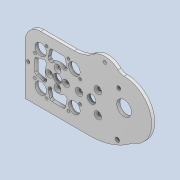
# Autodesk Inventor part: アームモータマウント
Saved by Autodesk Inventor 2020.4 (Build 244396000, 396)
## iProperties
Created: 2021-04-23
Part Number: アームモータマウント
Material: アルミニウム 2014-T4
Document SubType Name: Modeling
Designer: happy
Density: 2.8 g/cm^3
Appearance: サテン
Mass: 49.3876 g
Surface Area: 145.773 cm^2
Volume: 17.6384 cm^3
Author: happy
Autodesk Inventor part; units mm, degrees
ref_plane "YZ Plane" through (0, 0, 0) normal (1, 0, 0) x (0, 1, 0)
ref_plane "XZ Plane" through (0, 0, 0) normal (0, 1, 0) x (-1, 0, 0)
ref_plane "XY Plane" through (0, 0, 0) normal (0, 0, 1) x (1, 0, 0)
sketch "スケッチ1" plane through (0, 0, 0) normal (0, 0, 1) x (1, 0, 0)
  circle A0 centre (80.0196, 33.6804) radius 15
  circle A1 centre (112.2, 33.6804) radius 15
  circle A2 centre (112.2, 1.5) radius 15 construction
  circle A3 centre (80.0196, 1.5) radius 15 construction
  circle A4 centre (96.1098, 17.5902) radius 3.5 construction
  circle A5 centre (80.0196, 33.6804) radius 5.5
  circle A6 centre (112.2, 33.6804) radius 5.5
  circle A7 centre (80.0196, 1.5) radius 5.5
  circle A8 centre (112.2, 1.5) radius 5.5
  circle A9 centre (96.1098, 17.5902) radius 4.025
  circle A10 centre (74.3628, 28.0235) radius 1.3
  circle A11 centre (85.6765, 39.3372) radius 1.3
  circle A12 centre (106.5431, 39.3372) radius 1.3
  circle A13 centre (117.8569, 28.0235) radius 1.3
  circle A14 centre (117.8569, 7.1569) radius 1.3
  circle A15 centre (106.5431, -4.1569) radius 1.3
  circle A16 centre (85.6765, -4.1569) radius 1.3
  circle A17 centre (74.3628, 7.1569) radius 1.3
  line L0 (85.6765, 39.3372) -> (74.3628, 28.0235) construction
  line L1 (74.3628, 7.1569) -> (85.6765, -4.1569) construction
  line L2 (106.5431, -4.1569) -> (117.8569, 7.1569) construction
  line L3 (117.8569, 28.0235) -> (106.5431, 39.3372) construction
  line L4 (80.0196, 33.6804) -> (96.1098, 17.5902) construction
  line L5 (96.1098, 17.5902) -> (112.2, 33.6804) construction
  line L6 (112.2, 1.5) -> (96.1098, 17.5902) construction
  line L7 (80.0196, 1.5) -> (96.1098, 17.5902) construction
  circle A18 centre (74.3628, 28.0235) radius 3.3
  circle A19 centre (80.0196, 33.6804) radius 7.5
  circle A20 centre (85.6765, 39.3372) radius 3.3
  circle A21 centre (106.5431, 39.3372) radius 3.3
  circle A22 centre (112.2, 33.6804) radius 7.5
  circle A23 centre (117.8569, 28.0235) radius 3.3
  circle A24 centre (117.8569, 7.1569) radius 3.3
  circle A25 centre (112.2, 1.5) radius 7.5
  circle A26 centre (106.5431, -4.1569) radius 3.3
  circle A27 centre (85.6765, -4.1569) radius 3.3
  circle A28 centre (80.0196, 1.5) radius 7.5
  circle A29 centre (74.3628, 7.1569) radius 3.3
  line L8 (72.7217, 35.4098) -> (71.1517, 28.7845)
  line L9 (75.1237, 24.8125) -> (81.749, 26.3825)
  line L10 (87.3175, 31.951) -> (88.8875, 38.5763)
  line L11 (84.9155, 42.5483) -> (78.2902, 40.9783)
  line L12 (107.3041, 42.5483) -> (113.9294, 40.9783)
  line L13 (119.4979, 35.4098) -> (121.0679, 28.7845)
  line L14 (117.0959, 24.8125) -> (110.4706, 26.3825)
  line L15 (104.9021, 31.951) -> (103.3321, 38.5763)
  line L16 (121.0679, 6.3959) -> (119.4979, -0.2294)
  line L17 (110.4706, 8.7979) -> (117.0959, 10.3679)
  line L18 (104.9021, 3.2294) -> (103.3321, -3.3959)
  line L19 (113.9294, -5.7979) -> (107.3041, -7.3679)
  line L20 (71.1517, 6.3959) -> (72.7217, -0.2294)
  line L21 (78.2902, -5.7979) -> (84.9155, -7.3679)
  line L22 (88.8875, -3.3959) -> (87.3175, 3.2294)
  line L23 (81.749, 8.7979) -> (75.1237, 10.3679)
  circle A30 centre (96.1098, 25.6116) radius 3 construction
  circle A31 centre (104.1312, 17.5902) radius 3 construction
  circle A32 centre (96.1098, 9.5688) radius 3 construction
  circle A33 centre (88.0884, 17.5902) radius 3 construction
  circle A34 centre (96.1098, 25.6116) radius 1.25
  circle A35 centre (88.0884, 17.5902) radius 1.25
  circle A36 centre (96.1098, 9.5688) radius 1.25
  circle A37 centre (104.1312, 17.5902) radius 1.25
  circle A38 centre (96.1098, 17.5902) radius 12.0214
  circle A39 centre (96.1098, 25.6116) radius 4 construction
  line L24 (80.0196, 33.6804) -> (112.2, 33.6804) construction
  line L25 (112.2, 1.5) -> (112.2, 33.6804) construction
  line L26 (80.0196, 33.6804) -> (80.0196, 1.5) construction
  line L27 (80.0196, 1.5) -> (112.2, 1.5) construction
  line L28 (80.0196, 48.6804) -> (112.2, 48.6804)
  line L29 (127.2, 33.6804) -> (127.2, -14.5)
  line L30 (127.2, -14.5) -> (65.0196, -14.5)
  line L31 (65.0196, -14.5) -> (65.0196, 33.6804)
  line L32 (83, -14.5) -> (133, -14.5) construction
  line L33 (117.8569, 39.3372) -> (74.3628, 39.3372)
  line L34 (74.3628, 39.3372) -> (74.3628, -4.1569)
  line L35 (74.3628, -4.1569) -> (117.8569, -4.1569)
  line L36 (117.8569, -4.1569) -> (117.8569, 39.3372)
  line L37 (83.7167, 27.1549) -> (86.3137, 24.5579)
  line L38 (89.1421, 27.3863) -> (86.5451, 29.9833)
  line L39 (105.6745, 29.9833) -> (103.0775, 27.3863)
  line L40 (108.503, 27.1549) -> (105.9059, 24.5579)
  line L41 (108.503, 8.0255) -> (105.9059, 10.6225)
  line L42 (105.6745, 5.197) -> (103.0775, 7.7941)
  line L43 (83.7167, 8.0255) -> (86.3137, 10.6225)
  line L44 (86.5451, 5.197) -> (89.1421, 7.7941)
  circle A40 centre (96.1098, 45.6804) radius 3 construction
  circle A41 centre (68.0196, 17.5902) radius 3 construction
  circle A42 centre (68.0196, 17.5902) radius 1.5
  circle A43 centre (96.1098, 45.6804) radius 1.5
  line L45 (127.2, 33.6804) -> (127.2, -14.5) construction
  line L46 (83, -14.5) -> (133, -14.5) construction
  circle A44 centre (128.7687, 16.8502) radius 6.025 construction
  circle A45 centre (160, 25) radius 2
  circle A46 centre (154.8697, 39.0954) radius 1.75
  circle A47 centre (128.7687, 16.8502) radius 4.025
  arc A48 (112.2, 48.6804) -> (130.0806, 54.5913) centre (112.2, 78.6804) ccw
  arc A49 (153.3164, 53.0826) -> (130.0806, 54.5913) centre (140.809, 40.1379) ccw
  arc A50 (153.3164, 53.0826) -> (160, 50.3812) centre (160, 60) ccw
  arc A51 (168.6809, 1.1495) -> (160, 50.3812) centre (160, 25) ccw
  arc A52 (168.6809, 1.1495) -> (165.807, -0.5048) centre (171.9707, -7.8892) ccw
  arc A53 (127.2, -14.5) -> (165.807, -0.5048) centre (127.2, 45.748) ccw
  circle A54 centre (134.7937, 27.2858) radius 1.5
  circle A55 centre (116.7187, 16.8502) radius 1.5
  circle A56 centre (134.7937, 6.4146) radius 1.5
  circle A57 centre (160, 25) radius 7.025
  line L47 (65.0196, -14.5) -> (65.0196, 33.6804)
  circle A58 centre (80.0196, 33.6804) radius 15 construction
  line L48 (80.0196, 48.6804) -> (112.2, 48.6804)
  circle A59 centre (112.2, 33.6804) radius 15 construction
  line L49 (127.2, -14.5) -> (65.0196, -14.5)
  circle A60 centre (80.0196, 33.6804) radius 3.05 construction
  circle A61 centre (112.2, 33.6804) radius 3.05 construction
  circle A62 centre (112.2, 1.5) radius 3.05 construction
  circle A63 centre (80.0196, 1.5) radius 3.05 construction
  circle A64 centre (96.1098, 17.5902) radius 2.85 construction
  circle A65 centre (128.7687, 16.8502) radius 5.7 construction
  circle A66 centre (160, 25) radius 21.5 construction
  circle A67 centre (128.7687, 16.8502) radius 28.5 construction
  circle A68 centre (128.7687, 16.8502) radius 29.4672 construction
  circle A69 centre (160, 25) radius 25.8772 construction
  circle A70 centre (80.0196, 33.6804) radius 6
  circle A71 centre (112.2, 33.6804) radius 6
  circle A72 centre (80.0196, 1.5) radius 6
  circle A73 centre (112.2, 1.5) radius 6
  arc A74 (112.2, 48.6804) -> (130.3338, 54.7813) centre (112.2, 78.6804) ccw
  arc A75 (153.6832, 53.4235) -> (160, 50.8812) centre (160, 60) ccw
  arc A76 (153.6832, 53.4235) -> (130.3338, 54.7813) centre (141.2141, 40.4419) ccw
  circle A77 centre (96.1098, 17.5902) radius 9.025
  circle A78 centre (128.7687, 16.8502) radius 6.025
  circle A79 centre (160, 25) radius 2
  arc A80 (168.8519, 0.6796) -> (160, 50.8812) centre (160, 25) ccw
  arc A81 (168.8519, 0.6796) -> (166.2672, -0.7743) centre (171.9707, -7.8892) ccw
  circle A82 centre (171.9707, -7.8892) radius 8.6188 construction
  arc A83 (127.2, -14.5) -> (166.2672, -0.7743) centre (127.2, 47.9609) ccw
  circle A84 centre (160, 60) radius 8.6188 construction
  circle A85 centre (154.8697, 39.0954) radius 3 construction
  circle A86 centre (154.8697, 39.0954) radius 1.75
  arc A87 (158.348, 26.1273) -> (99.1742, 26.079) centre (128.7687, 16.8502) ccw construction
  arc A88 (98.7866, 8.9713) -> (159.1095, 23.2092) centre (128.7687, 16.8502) ccw construction
  arc A89 (80.0196, 48.6804) -> (65.0196, 33.6804) centre (80.0196, 33.6804) ccw
  line L50 (65.0196, -14.5) -> (65.0196, 33.6804)
  circle A90 centre (80.0196, 33.6804) radius 15 construction
  line L51 (80.0196, 48.6804) -> (112.2, 48.6804)
  circle A91 centre (112.2, 33.6804) radius 15 construction
  line L52 (127.2, -14.5) -> (65.0196, -14.5)
  circle A92 centre (80.0196, 33.6804) radius 3.05 construction
  circle A93 centre (112.2, 33.6804) radius 3.05 construction
  circle A94 centre (112.2, 1.5) radius 3.05 construction
  circle A95 centre (80.0196, 1.5) radius 3.05 construction
  circle A96 centre (96.1098, 17.5902) radius 2.85 construction
  circle A97 centre (128.7687, 16.8502) radius 5.7 construction
  circle A98 centre (160, 25) radius 21.5 construction
  circle A99 centre (128.7687, 16.8502) radius 28.5 construction
  circle A100 centre (128.7687, 16.8502) radius 29.4672 construction
  circle A101 centre (160, 25) radius 25.8772 construction
  circle A102 centre (80.0196, 33.6804) radius 6
  circle A103 centre (112.2, 33.6804) radius 6
  circle A104 centre (80.0196, 1.5) radius 6
  circle A105 centre (112.2, 1.5) radius 6
  arc A106 (112.2, 48.6804) -> (130.5847, 54.9738) centre (112.2, 78.6804) ccw
  arc A107 (154.0473, 53.767) -> (160, 51.3812) centre (160, 60) ccw
  arc A108 (154.0473, 53.767) -> (130.5847, 54.9738) centre (141.6155, 40.7498) ccw
  circle A109 centre (96.1098, 17.5902) radius 9.025
  circle A110 centre (128.7687, 16.8502) radius 6.025
  circle A111 centre (160, 25) radius 2
  arc A112 (169.0229, 0.2098) -> (160, 51.3812) centre (160, 25) ccw
  arc A113 (169.0229, 0.2098) -> (166.7152, -1.0582) centre (171.9707, -7.8892) ccw
  circle A114 centre (171.9707, -7.8892) radius 8.6188 construction
  arc A115 (127.2, -14.5) -> (166.7152, -1.0582) centre (127.2, 50.3027) ccw
  circle A116 centre (160, 60) radius 8.6188 construction
  circle A117 centre (154.8697, 39.0954) radius 3 construction
  circle A118 centre (154.8697, 39.0954) radius 1.75
  arc A119 (158.348, 26.1273) -> (99.1742, 26.079) centre (128.7687, 16.8502) ccw construction
  arc A120 (98.7866, 8.9713) -> (159.1094, 23.2092) centre (128.7687, 16.8502) ccw construction
  arc A121 (80.0196, 48.6804) -> (65.0196, 33.6804) centre (80.0196, 33.6804) ccw
  circle A122 centre (141.6155, 53.7498) radius 5 construction
  circle A123 centre (141.6155, 53.7498) radius 3.2
  circle A124 centre (141.6155, 53.7498) radius 1.5
  circle A125 centre (153.5524, -4.4926) radius 2
  circle A126 centre (153.5524, -4.4926) radius 4 construction
  point P0 (0, 0)
  point P1 (0, 0)
  point P2 (117.8569, 24.7235)
  point P3 (117.8569, 10.4569)
  point P4 (103.2431, -4.1569)
  point P5 (88.9765, -4.1569)
  point P6 (88.9765, 39.3372)
  point P7 (103.2431, 39.3372)
  point P8 (74.3628, 10.4569)
  point P9 (74.3628, 24.7235)
  point P10 (167.1721, 0.4471)
  point P11 (0, 0)
  point P12 (96.1924, 17.5902)
  point P13 (80.1022, 1.5)
  point P14 (112.2826, 1.5)
  point P15 (112.2826, 33.6804)
  point P16 (80.1022, 33.6804)
  point P17 (160, 60)
  point P18 (147.9041, -10.9688)
  point P19 (0, 0)
  point P20 (96.1924, 17.5902)
  point P21 (80.1022, 1.5)
  point P22 (112.2826, 1.5)
  point P23 (112.2826, 33.6804)
  point P24 (80.1022, 33.6804)
  point P25 (160, 60)
  point P26 (148.0694, -11.0476)
  point P27 (130.3338, 54.7813)
  dimension "d0" = 11
  dimension "d1" = 2.6
  dimension "d2" = 16
  dimension "d3" = 2
  dimension "d4" = 2
  dimension "d5" = 2
  dimension "d6" = 8.05
  dimension "d7" = 6
  dimension "d8" = 2.5
  dimension "d9" = 8
  dimension "d10" = 4
  dimension "d11" = 4
  dimension "d12" = 4
  dimension "d13" = 4
  dimension "d14" = 6
  dimension "d15" = 6
  dimension "d16" = 3
  dimension "d17" = 3
  dimension "d21" = 8.05
  dimension "d22" = 3
  dimension "d36" = 14.05
  dimension "d38" = 12
  dimension "d39" = 30
  dimension "d40" = 18.05
  dimension "d41" = 12.05
  dimension "d42" = 4
  dimension "d43" = 0.5
  dimension "d44" = 18
  dimension "d45" = 3.5
  dimension "d46" = 31
  dimension "d47" = 62.4609
  dimension "d48" = 12
  dimension "d49" = 30
  dimension "d50" = 18.05
  dimension "d51" = 12.05
  dimension "d52" = 4
  dimension "d53" = 0
  dimension "d54" = 18
  dimension "d55" = 3.5
  dimension "d56" = 31
  dimension "d57" = 64.8027
  dimension "d58" = 10
  dimension "d59" = 6.4
  dimension "d60" = 3
  dimension "d68" = 4
  dimension "d69" = 8
  constraints: 122 centre point, 106 end point, 103 point on circle, 64 tangent, 40 coincident, 36 equal radius, 9 parallel, 6 concentric, 5 perpendicular, 5 vertical alignment, 4 horizontal, 4 midpoint, 3 equal length, 2 point on line, 2 vertical, 1 horizontal alignment, 50 other
  measures "d0" diameter of A5
  measures "d1" diameter of A10
  measures "d2" distance of L0.start L0.end
  measures "d3" radial gap between concentric circles of A10 A18
  measures "d4" radial gap between concentric circles of A5 A19
  measures "d5" radial gap between concentric circles of A11 A20
  measures "d6" diameter of A9
  measures "d7" diameter of A30
  measures "d8" diameter of A34
  measures "d9" diameter of A39
  measures "d10" distance between parallel lines of L37 L38
  measures "d11" distance between parallel lines of L40 L39
  measures "d12" distance between parallel lines of L42 L41
  measures "d13" distance between parallel lines of L44 L43
  measures "d14" diameter of A40
  measures "d15" diameter of A41
  measures "d16" diameter of A42
  measures "d17" diameter of A43
  measures "d21" diameter of A47
  measures "d22" diameter of A54
  measures "d36" diameter of A57
  measures "d38" diameter of A71
  measures "d39" radius of A74
  measures "d40" diameter of A77
  measures "d41" diameter of A78
  measures "d42" diameter of A79
  measures "d43" radial gap between concentric circles of A82 A81
  measures "d44" radius of A76
  measures "d45" diameter of A86
  measures "d46" radius of A87
  measures "d47" radius of A83
  measures "d48" diameter of A103
  measures "d49" radius of A106
  measures "d50" diameter of A109
  measures "d51" diameter of A110
  measures "d52" diameter of A111
  measures "d53" radial gap between concentric circles of A114 A113
  measures "d54" radius of A108
  measures "d55" diameter of A118
  measures "d56" radius of A119
  measures "d57" radius of A115
  measures "d58" diameter of A122
  measures "d59" diameter of A123
  measures "d60" diameter of A124
  measures "d68" diameter of A125
  measures "d69" diameter of A126
extrude "押し出し1" add sketch "スケッチ1" along normal blind 3 contours A0 L33 A20 L11 A19 L34 L8 A18 | L28 A1 L33 A0 | A0 L34 A29 L20 A28 L35 L21 A27 A26 L19 A25 L36 L16 A24 A55 A1 L29 A78 L30 L31 | A48 A49 A50 A51 A52 A53 L29 A78 A1 | A1 L36 A23 L13 A22 L33 L12 A21 | L33 A11 A19 A20 | A20 A19 A11 L33 | A74 A76 A75 A80 A81 A83 A53 A52 A51 A50 A49 | A38 A0 A77 | A0 A77 A35 A36 A37 A1 A38 | L34 A10 A19 A18 | A18 A19 A10 L34 | L34 A17 A28 A29 | A29 A28 A17 L34 | A83 A81 A80 A75 A76 A106 A108 A107 A112 A113 A115 | A38 A1 A77 A34 A0 | A38 A1 A77 | L33 A12 A22 A21 | A21 A22 A12 L33 | A20 A19 L11 | L10 A19 A20 | L36 A55 A24 L17 A25 L41 A38 A1 | A1 A38 L40 A22 L14 A23 L36 | A78 L29 A47 | L29 A47 A78 | A77 A0 | A0 A77 A34 A1 A37 A36 A35 | L37 A19 L38 A38 | A38 L44 A28 L43 | L8 A19 A18 | A18 A19 L9 | L23 A28 A29 | A29 A28 L20 | A77 A1 | L39 A22 L40 A38 | L12 A22 A21 | A21 A22 L15 | A20 L33 A70 A19 | A19 A11 L33 A20 | A20 A70 L33 A11 A19 | A19 A18 A70 A20 | L36 A13 A22 A23 | A23 A22 A13 L36 | A28 A27 A72 A29 | A19 L34 A70 A18 | A18 L34 A10 A19 | A19 A10 L34 A18 A70 | A29 A72 L34 A17 A28 | A29 L34 A72 A28 | A28 A17 L34 A29 | A22 A21 A71 A23 | A22 L33 A71 A21 | A21 L33 A12 A22 | A22 A12 L33 A21 A71 | A20 A70 L33 | L33 A70 L34 A19 | A19 L34 L33 | A70 A18 A5 A20 | A20 A5 A70 | L14 A22 A23 | A38 L41 A25 L42 | L34 A70 A18 | A29 A72 L34 | L34 A72 L35 A28 | A28 L35 L34 | L33 A71 A21 | L33 L36 A22 | A22 L36 A71 L33 | A71 A21 A6 | A21 A6 A23 A71 | A20 A5 A18 A70 L34 L33 | L33 A70 | L36 A14 A25 A24 | A24 A25 A14 L36 | A23 A71 L36 A13 A22 | A23 A22 L13 | A25 A24 A73 A26 | L22 A27 A28 | A18 A5 A70 | A70 L34 | A72 A27 A7 A29 | A29 A7 A72 | A29 A7 A27 A72 L35 L34 | L34 A72 | L35 A72 A27 A28 | A71 L33 L36 A23 A6 A21 | A71 L33 | A22 A23 L36 A71 | A23 A6 A71 | A24 A25 L17 | A22 A13 L36 A23 | A25 A26 L18 | A27 L35 A16 A28 | A28 A27 L21 | L35 A72 | A71 L36 | A71 L36 A23 | L16 A25 A24 | A25 A14 L36 A24 A73 | A26 A73 L35 A15 A25 | A25 A15 L35 A26 | A28 A16 L35 A27 A72 | A27 A28 A16 L35 | A72 A27 A7 | A27 L35 A16 A28 | A72 A27 L35 | A25 L36 A73 A24 | A24 L36 A14 A25 | A73 A24 A8 | A24 A8 A26 A73 | A26 A8 A73 | L35 A15 A25 A26 | L36 A73 A24 | L36 L35 A25 | A25 L35 A73 L36 | A73 L36 L35 A26 A8 A24 | L35 A26 A25 A15 | A73 L35 A26 | A26 A25 L19 | A73 L36 | A25 A26 L35 A73 | L35 A73 | A43 | A123 | A124 | A125
fillet "フィレット1" radius 2 18 edges at (86.5451, 5.197, 1.5) (89.1421, 7.7941, 1.5) (88.9765, -4.1569, 1.5) (103.2431, -4.1569, 1.5) (105.6745, 5.197, 1.5) (103.0775, 7.7941, 1.5) (103.0775, 27.3863, 1.5) (105.6745, 29.9833, 1.5) (103.2431, 39.3372, 1.5) (88.9765, 39.3372, 1.5) (86.5451, 29.9833, 1.5) (89.1421, 27.3863, 1.5) (83.7167, 27.1549, 1.5) (74.3628, 24.7235, 1.5) (86.3137, 24.5579, 1.5) (74.3628, 10.4569, 1.5) (83.7167, 8.0255, 1.5) (86.3137, 10.6225, 1.5)
chamfer "面取り1" distance 2 angle 45 7 edges at (115.2187, 16.8502, 3) (133.2937, 27.2858, 3) (133.2937, 6.4146, 3) (94.8598, 25.6116, 3) (86.8384, 17.5902, 3) (94.8598, 9.5688, 3) (102.8812, 17.5902, 3)
sketch "スケッチ2" plane through (0, 0, 0) normal (0, 0, -1) x (-1, 0, 0)
  line L0 (-81.749, 8.7979) -> (-75.9016, 10.1836) projected
  arc A0 (-81.749, 8.7979) -> (-82.5969, 8.5433) centre (-80.0196, 1.5) ccw projected
  arc A1 (-84.6984, 9.0072) -> (-82.5969, 8.5433) centre (-83.2842, 10.4215) ccw projected
  line L1 (-85.193, 9.5018) -> (-84.6984, 9.0072) projected
  arc A2 (-85.5377, 11.868) -> (-85.193, 9.5018) centre (-83.7788, 10.916) ccw projected
  arc A3 (-85.5377, 11.868) -> (-85.5377, 23.3124) centre (-96.1098, 17.5902) ccw projected
  arc A4 (-85.193, 25.6786) -> (-85.5377, 23.3124) centre (-83.7788, 24.2644) ccw projected
  line L2 (-84.6984, 26.1731) -> (-85.193, 25.6786) projected
  arc A5 (-82.5969, 26.6371) -> (-84.6984, 26.1731) centre (-83.2842, 24.7589) ccw projected
  arc A6 (-82.5969, 26.6371) -> (-81.749, 26.3825) centre (-80.0196, 33.6804) ccw projected
  line L3 (-75.9016, 24.9968) -> (-81.749, 26.3825) projected
  arc A7 (-74.3628, 23.0507) -> (-75.9016, 24.9968) centre (-76.3628, 23.0507) ccw projected
  line L4 (-74.3628, 12.1297) -> (-74.3628, 23.0507) projected
  arc A8 (-75.9016, 10.1836) -> (-74.3628, 12.1297) centre (-76.3628, 12.1297) ccw projected
  line L5 (-65.0196, 33.6804) -> (-65.0196, -14.5) projected
  arc A9 (-65.0196, 33.6804) -> (-80.0196, 48.6804) centre (-80.0196, 33.6804) ccw projected
  line L6 (-112.2, 48.6804) -> (-80.0196, 48.6804) projected
  line L7 (-65.0196, -14.5) -> (-127.2, -14.5) projected
  circle A10 centre (-74.3628, 28.0235) radius 1.3 projected
  circle A11 centre (-112.2, 33.6804) radius 5.5 projected
  circle A12 centre (-80.0196, 1.5) radius 5.5 projected
  circle A13 centre (-112.2, 1.5) radius 5.5 projected
  circle A14 centre (-80.0196, 33.6804) radius 5.5 projected
  line L8 (-104.9021, 3.2294) -> (-103.5164, -2.618) projected
  arc A15 (-104.9021, 3.2294) -> (-105.1567, 4.0773) centre (-112.2, 1.5) ccw projected
  arc A16 (-104.6928, 6.1788) -> (-105.1567, 4.0773) centre (-103.2785, 4.7646) ccw projected
  line L9 (-104.1982, 6.6734) -> (-104.6928, 6.1788) projected
  arc A17 (-101.832, 7.0181) -> (-104.1982, 6.6734) centre (-102.784, 5.2592) ccw projected
  arc A18 (-101.832, 7.0181) -> (-90.3876, 7.0181) centre (-96.1098, 17.5902) ccw projected
  arc A19 (-88.0214, 6.6734) -> (-90.3876, 7.0181) centre (-89.4356, 5.2592) ccw projected
  line L10 (-87.5269, 6.1788) -> (-88.0214, 6.6734) projected
  arc A20 (-87.0629, 4.0773) -> (-87.5269, 6.1788) centre (-88.9411, 4.7646) ccw projected
  arc A21 (-87.0629, 4.0773) -> (-87.3175, 3.2294) centre (-80.0196, 1.5) ccw projected
  line L11 (-88.7032, -2.618) -> (-87.3175, 3.2294) projected
  arc A22 (-90.6493, -4.1569) -> (-88.7032, -2.618) centre (-90.6493, -2.1569) ccw projected
  line L12 (-101.5703, -4.1569) -> (-90.6493, -4.1569) projected
  arc A23 (-103.5164, -2.618) -> (-101.5703, -4.1569) centre (-101.5703, -2.1569) ccw projected
  circle A24 centre (-74.3628, 7.1569) radius 1.3 projected
  circle A25 centre (-117.8569, 28.0235) radius 1.3 projected
  circle A26 centre (-106.5431, -4.1569) radius 1.3 projected
  circle A27 centre (-117.8569, 7.1569) radius 1.3 projected
  circle A28 centre (-128.7687, 16.8502) radius 4.025 projected
  circle A29 centre (-154.8697, 39.0954) radius 1.75 projected
  circle A30 centre (-134.7937, 27.2858) radius 1.5 projected
  circle A31 centre (-134.7937, 6.4146) radius 1.5 projected
  circle A32 centre (-68.0196, 17.5902) radius 1.5 projected
  circle A33 centre (-116.7187, 16.8502) radius 1.5 projected
  circle A34 centre (-104.1312, 17.5902) radius 1.25 projected
  circle A35 centre (-96.1098, 9.5688) radius 1.25 projected
  circle A36 centre (-88.0884, 17.5902) radius 1.25 projected
  circle A37 centre (-96.1098, 25.6116) radius 1.25 projected
  circle A38 centre (-96.1098, 17.5902) radius 4.025 projected
  circle A39 centre (-85.6765, -4.1569) radius 1.3 projected
  circle A40 centre (-106.5431, 39.3372) radius 1.3 projected
  circle A41 centre (-85.6765, 39.3372) radius 1.3 projected
  line L13 (-87.3175, 31.951) -> (-88.7032, 37.7984) projected
  arc A42 (-87.3175, 31.951) -> (-87.0629, 31.1031) centre (-80.0196, 33.6804) ccw projected
  arc A43 (-87.5269, 29.0016) -> (-87.0629, 31.1031) centre (-88.9411, 30.4158) ccw projected
  line L14 (-88.0214, 28.507) -> (-87.5269, 29.0016) projected
  arc A44 (-90.3876, 28.1623) -> (-88.0214, 28.507) centre (-89.4356, 29.9212) ccw projected
  arc A45 (-90.3876, 28.1623) -> (-101.832, 28.1623) centre (-96.1098, 17.5902) ccw projected
  arc A46 (-104.1982, 28.507) -> (-101.832, 28.1623) centre (-102.784, 29.9212) ccw projected
  line L15 (-104.6928, 29.0016) -> (-104.1982, 28.507) projected
  arc A47 (-105.1567, 31.1031) -> (-104.6928, 29.0016) centre (-103.2785, 30.4158) ccw projected
  arc A48 (-105.1567, 31.1031) -> (-104.9021, 31.951) centre (-112.2, 33.6804) ccw projected
  line L16 (-103.5164, 37.7984) -> (-104.9021, 31.951) projected
  arc A49 (-101.5703, 39.3372) -> (-103.5164, 37.7984) centre (-101.5703, 37.3372) ccw projected
  line L17 (-90.6493, 39.3372) -> (-101.5703, 39.3372) projected
  arc A50 (-88.7032, 37.7984) -> (-90.6493, 39.3372) centre (-90.6493, 37.3372) ccw projected
  circle A51 centre (-68.0196, 17.5902) radius 1.5 projected
  circle A52 centre (-68.0196, 17.5902) radius 3.025
  arc A53 (-130.5847, 54.9738) -> (-112.2, 48.6804) centre (-112.2, 78.6804) ccw projected
  arc A54 (-130.5847, 54.9738) -> (-154.0473, 53.767) centre (-141.6155, 40.7498) ccw projected
  arc A55 (-160, 51.3812) -> (-154.0473, 53.767) centre (-160, 60) ccw projected
  arc A56 (-160, 51.3812) -> (-169.0229, 0.2098) centre (-160, 25) ccw projected
  arc A57 (-166.7152, -1.0582) -> (-169.0229, 0.2098) centre (-171.9707, -7.8892) ccw projected
  arc A58 (-166.7152, -1.0582) -> (-127.2, -14.5) centre (-127.2, 50.3027) ccw projected
  point P0 (0, 0)
  point P1 (-65.0196, 17.2021)
  point P2 (-65.0196, 17.9783)
  dimension "d26" = 6.05
  constraints: 1 centre point, 1 coincident
  measures "d26" diameter of A52
extrude "押し出し2" cut sketch "スケッチ2" against normal blind 1 contours L5 A52 picked at (-65.5196, 17.5902)
fillet "フィレット2" radius 1 2 edges at (65.0196, 17.9783, 0.5) (65.0196, 17.2021, 0.5)
sketch "スケッチ3" plane through (0, 0, 3) normal (0, 0, 1) x (1, 0, 0)
  circle A0 centre (96.1098, 9.5688) radius 3.25 projected
  circle A1 centre (96.1098, 25.6116) radius 3.25 projected
  circle A2 centre (134.7937, 27.2858) radius 3.5 projected
  line L0 (65.0196, 33.6804) -> (65.0196, -14.5) projected
  line L1 (65.0196, -14.5) -> (127.2, -14.5) projected
  arc A3 (127.2, -14.5) -> (166.7152, -1.0582) centre (127.2, 50.3027) ccw projected
  arc A4 (169.0229, 0.2098) -> (166.7152, -1.0582) centre (171.9707, -7.8892) ccw projected
  arc A5 (169.0229, 0.2098) -> (160, 51.3812) centre (160, 25) ccw projected
  arc A6 (154.0473, 53.767) -> (160, 51.3812) centre (160, 60) ccw projected
  arc A7 (154.0473, 53.767) -> (130.5847, 54.9738) centre (141.6155, 40.7498) ccw projected
  arc A8 (112.2, 48.6804) -> (130.5847, 54.9738) centre (112.2, 78.6804) ccw projected
  line L2 (112.2, 48.6804) -> (80.0196, 48.6804) projected
  arc A9 (80.0196, 48.6804) -> (65.0196, 33.6804) centre (80.0196, 33.6804) ccw projected
  circle A10 centre (80.0196, 33.6804) radius 5.5 projected
  circle A11 centre (112.2, 33.6804) radius 5.5 projected
  circle A12 centre (74.3628, 7.1569) radius 1.3 projected
  circle A13 centre (112.2, 1.5) radius 5.5 projected
  circle A14 centre (74.3628, 28.0235) radius 1.3 projected
  circle A15 centre (117.8569, 28.0235) radius 1.3 projected
  circle A16 centre (68.0196, 17.5902) radius 1.5 projected
  circle A17 centre (128.7687, 16.8502) radius 4.025 projected
  circle A18 centre (154.8697, 39.0954) radius 1.75 projected
  circle A19 centre (160, 25) radius 7.025 projected
  circle A20 centre (96.1098, 17.5902) radius 4.025 projected
  circle A21 centre (117.8569, 7.1569) radius 1.3 projected
  circle A22 centre (85.6765, -4.1569) radius 1.3 projected
  line L3 (104.9021, 3.2294) -> (103.5164, -2.618) projected
  arc A23 (101.5703, -4.1569) -> (103.5164, -2.618) centre (101.5703, -2.1569) ccw projected
  line L4 (101.5703, -4.1569) -> (90.6493, -4.1569) projected
  arc A24 (88.7032, -2.618) -> (90.6493, -4.1569) centre (90.6493, -2.1569) ccw projected
  line L5 (88.7032, -2.618) -> (87.3175, 3.2294) projected
  arc A25 (87.3175, 3.2294) -> (87.0629, 4.0773) centre (80.0196, 1.5) ccw projected
  arc A26 (87.5269, 6.1788) -> (87.0629, 4.0773) centre (88.9411, 4.7646) ccw projected
  line L6 (87.5269, 6.1788) -> (88.0214, 6.6734) projected
  arc A27 (90.3876, 7.0181) -> (88.0214, 6.6734) centre (89.4356, 5.2592) ccw projected
  arc A28 (90.3876, 7.0181) -> (101.832, 7.0181) centre (96.1098, 17.5902) ccw projected
  arc A29 (104.1982, 6.6734) -> (101.832, 7.0181) centre (102.784, 5.2592) ccw projected
  line L7 (104.1982, 6.6734) -> (104.6928, 6.1788) projected
  arc A30 (105.1567, 4.0773) -> (104.6928, 6.1788) centre (103.2785, 4.7646) ccw projected
  arc A31 (105.1567, 4.0773) -> (104.9021, 3.2294) centre (112.2, 1.5) ccw projected
  circle A32 centre (106.5431, -4.1569) radius 1.3 projected
  circle A33 centre (106.5431, 39.3372) radius 1.3 projected
  circle A34 centre (85.6765, 39.3372) radius 1.3 projected
  line L8 (87.3175, 31.951) -> (88.7032, 37.7984) projected
  arc A35 (90.6493, 39.3372) -> (88.7032, 37.7984) centre (90.6493, 37.3372) ccw projected
  line L9 (90.6493, 39.3372) -> (101.5703, 39.3372) projected
  arc A36 (103.5164, 37.7984) -> (101.5703, 39.3372) centre (101.5703, 37.3372) ccw projected
  line L10 (103.5164, 37.7984) -> (104.9021, 31.951) projected
  arc A37 (104.9021, 31.951) -> (105.1567, 31.1031) centre (112.2, 33.6804) ccw projected
  arc A38 (104.6928, 29.0016) -> (105.1567, 31.1031) centre (103.2785, 30.4158) ccw projected
  line L11 (104.6928, 29.0016) -> (104.1982, 28.507) projected
  arc A39 (101.832, 28.1623) -> (104.1982, 28.507) centre (102.784, 29.9212) ccw projected
  arc A40 (101.832, 28.1623) -> (90.3876, 28.1623) centre (96.1098, 17.5902) ccw projected
  arc A41 (88.0214, 28.507) -> (90.3876, 28.1623) centre (89.4356, 29.9212) ccw projected
  line L12 (88.0214, 28.507) -> (87.5269, 29.0016) projected
  arc A42 (87.0629, 31.1031) -> (87.5269, 29.0016) centre (88.9411, 30.4158) ccw projected
  arc A43 (87.0629, 31.1031) -> (87.3175, 31.951) centre (80.0196, 33.6804) ccw projected
  circle A44 centre (80.0196, 1.5) radius 5.5 projected
  line L13 (75.9016, 24.9968) -> (81.749, 26.3825) projected
  arc A45 (81.749, 26.3825) -> (82.5969, 26.6371) centre (80.0196, 33.6804) ccw projected
  arc A46 (84.6984, 26.1731) -> (82.5969, 26.6371) centre (83.2842, 24.7589) ccw projected
  line L14 (84.6984, 26.1731) -> (85.193, 25.6786) projected
  arc A47 (85.5377, 23.3124) -> (85.193, 25.6786) centre (83.7788, 24.2644) ccw projected
  arc A48 (85.5377, 23.3124) -> (85.5377, 11.868) centre (96.1098, 17.5902) ccw projected
  arc A49 (85.193, 9.5018) -> (85.5377, 11.868) centre (83.7788, 10.916) ccw projected
  line L15 (85.193, 9.5018) -> (84.6984, 9.0072) projected
  arc A50 (82.5969, 8.5433) -> (84.6984, 9.0072) centre (83.2842, 10.4215) ccw projected
  arc A51 (82.5969, 8.5433) -> (81.749, 8.7979) centre (80.0196, 1.5) ccw projected
  line L16 (81.749, 8.7979) -> (75.9016, 10.1836) projected
  arc A52 (74.3628, 12.1297) -> (75.9016, 10.1836) centre (76.3628, 12.1297) ccw projected
  line L17 (74.3628, 12.1297) -> (74.3628, 23.0507) projected
  arc A53 (75.9016, 24.9968) -> (74.3628, 23.0507) centre (76.3628, 23.0507) ccw projected
  circle A54 centre (116.7187, 16.8502) radius 3.5 projected
  circle A55 centre (134.7937, 6.4146) radius 3.5 projected
  circle A56 centre (88.0884, 17.5902) radius 3.25 projected
  circle A57 centre (104.1312, 17.5902) radius 3.25 projected
  circle A58 centre (141.6155, 53.7498) radius 1.5 projected
  point P0 (0, 0)
extrude "押し出し3" cut sketch "スケッチ3" against normal blind 10 contours A58
extrude "押し出し4" cut sketch "スケッチ1" along normal blind 1 contours A123
extrude "押し出し5" cut sketch "スケッチ1" along normal blind 10 contours A125
equation "\"d11\" = d10"
equation "\"d12\" = d10"
equation "\"d13\" = d10"
